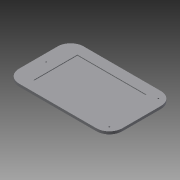
# Autodesk Inventor part: sensor_board_base
Saved by Autodesk Inventor 2013 (Build 170138000, 138)
## iProperties
Created: 2013-08-09
Part Number: sensor_board_base
Material: Generic
Document SubType Name: Modeling
Designer: Marc Bucchieri
Density: 1 g/cm^3
Author: Marc Bucchieri
Autodesk Inventor part; units mm, degrees
ref_plane "YZ Plane" through (0, 0, 0) normal (1, 0, 0) x (0, 1, 0)
ref_plane "XZ Plane" through (0, 0, 0) normal (0, 1, 0) x (-1, 0, 0)
ref_plane "XY Plane" through (0, 0, 0) normal (0, 0, 1) x (1, 0, 0)
sketch "Sketch1" plane through (0, 0, 0) normal (0, 1, 0) x (-1, 0, 0)
  line L0 (50.8, -31.75) -> (-50.8, -31.75)
  line L1 (-50.8, -31.75) -> (-50.8, 31.75)
  line L2 (-50.8, 31.75) -> (50.8, 31.75)
  line L3 (50.8, 31.75) -> (50.8, -31.75)
  line L4 (-57.1863, 0) -> (79.611, 0) construction
  point P0 (0, 0)
  dimension "d0" = 63.5
  dimension "d2" = 101.6
  dimension "d25" = 31.75
  dimension "d36" = 50.8
  constraints: 10 end point, 2 horizontal, 2 parallel, 2 perpendicular
  measures "d0" distance of L2.end L0.start
  measures "d2" distance of L0.start L0.end
  measures "d25" distance between parallel lines of L2 L4
  measures "d36" distance from line of L1 point (0, 0)
extrude "Extrusion1" add sketch "Sketch1" along normal blind 2.54
sketch "Sketch2" plane through (0, 0, 0) normal (0, -1, 0) x (1, 0, 0)
  line L0 (-50.8, -31.75) -> (50.8, -31.75) projected
  line L1 (50.8, -31.75) -> (50.8, 31.75) projected
  line L2 (50.8, 31.75) -> (-50.8, 31.75) projected
  line L3 (-50.8, 31.75) -> (-50.8, -31.75) projected
  circle A0 centre (-43.18, 0) radius 3.175
  circle A1 centre (43.18, 24.13) radius 3.175
  circle A2 centre (43.18, -24.13) radius 3.175
  line L4 (43.18, 24.13) -> (43.18, -24.13) construction
  point P0 (0, 0)
  dimension "d5" = 6.35
  dimension "d6" = 7.62
  dimension "d7" = 6.35
  dimension "d8" = 7.62
  dimension "d9" = 7.62
  dimension "d12" = 6.35
  dimension "d13" = 7.62
  dimension "d26" = 31.75
  constraints: 5 coincident, 3 centre point, 2 end point, 1 vertical
  measures "d5" diameter of A0
  measures "d6" distance from line of L3 A0.centre
  measures "d7" diameter of A1
  measures "d8" distance from line of L1 A1.centre
  measures "d9" distance from line of L2 A1.centre
  measures "d12" diameter of A2
  measures "d13" distance from line of L0 L4.end
  measures "d26" distance from line of L2 point (-43.18, 0)
extrude "Extrusion2" add sketch "Sketch2" along normal blind 2.032 contours A0 | A1 | A2
hole "Hole1" at (43.18, -2.032, 24.13) direction (0, 1, 0) diameter 1.27 end through all
mirror "Mirror1" about plane through (0, 0, 0) normal (0, 0, 1) of "Hole1"
sketch "Sketch4" plane through (-43.18, -2.032, 0) normal (0, -1, 0) x (1, 0, 0)
  circle A0 centre (0, 0) radius 3.175 projected
  point P0 (43.18, 0)
  constraints: 2 coincident
hole "Hole2" at (-43.18, -2.032, 0) direction (0, 1, 0) diameter 1.27 end through all
sketch "Sketch5" plane through (0, 2.54, 0) normal (0, 1, 0) x (1, 0, 0)
  line L0 (-33.9981, 21.59) -> (33.797, 21.59)
  line L1 (33.797, 21.59) -> (33.797, -21.59)
  line L2 (33.797, -21.59) -> (-33.9981, -21.59)
  line L3 (-33.9981, -21.59) -> (-33.9981, 21.59)
  point P0 (0, 0)
  constraints: 8 end point, 2 parallel, 1 horizontal, 1 perpendicular
extrude "Extrusion3" cut sketch "Sketch5" against normal blind 0.762
fillet "Fillet1" radius 12.7 4 edges at (-50.8, 1.27, 31.75) (50.8, 1.27, 31.75) (50.8, 1.27, -31.75) (-50.8, 1.27, -31.75)
chamfer "Chamfer1" distance 2.032 angle 45 3 edges at (40.005, 0, -24.13) (40.005, 0, 24.13) (-46.355, 0, 0)
equation "\"d6\" = d13"
equation "\"d8\" = d13"
body "Solid1"
